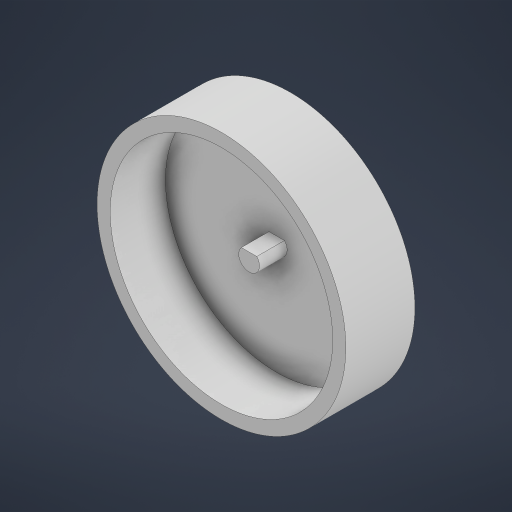
# Autodesk Inventor part: forma_do_kół
Saved by Autodesk Inventor 2023.4 (Build 274418000, 418)
## iProperties
Created: 2025-10-31
Part Number: forma_do_kół
Material: Ogólny
Document SubType Name: Modeling
Designer: Jakub Borsukiewicz
Density: 1 g/cm^3
Appearance: Domyślna
Author: Jakub Borsukiewicz
Autodesk Inventor part; units mm, degrees
ref_plane "YZ Plane" through (0, 0, 0) normal (1, 0, 0) x (0, 1, 0)
ref_plane "XZ Plane" through (0, 0, 0) normal (0, 1, 0) x (-1, 0, 0)
ref_plane "XY Plane" through (0, 0, 0) normal (0, 0, 1) x (1, 0, 0)
sketch "Szkic1" plane through (0, 0, 0) normal (0, 0, 1) x (1, 0, 0)
  circle A0 centre (0, 0) radius 18
  dimension "d0" = 36
  constraints: 1 centre point, 1 coincident
  measures "d0" diameter of A0
extrude "Wyciągnięcie proste1" add sketch "Szkic1" along normal blind 2
sketch "Szkic2" plane through (0, 0, 2) normal (0, 0, 1) x (1, 0, 0)
  circle A0 centre (0, 0) radius 1.5
  line L0 (0, 25.2) -> (0, -25.2) projected
  line L1 (-25.2, 0) -> (25.2, 0) projected
  line L2 (-1.118, 1) -> (1.118, 1)
  circle A1 centre (0, 0) radius 18 projected
  dimension "d3" = 3
  dimension "d4" = 1
  constraints: 2 end point, 2 point on circle, 1 centre point, 1 coincident, 1 horizontal
  measures "d3" diameter of A0
  measures "d4" distance between parallel lines of L1 L2
extrude "Wyciągnięcie proste2" add sketch "Szkic2" along normal blind 4 contours L1 L0 L2 A0 | A0 L0 L1 | A0 L1 L0 | L1 A0 L2 L0
sketch "Szkic3" plane through (0, 0, 2) normal (0, 0, 1) x (1, 0, 0)
  line L0 (-1.118, 1) -> (1.118, 1) projected
  arc A0 (-1.118, 1) -> (1.118, 1) centre (0, 0) ccw projected
  circle A1 centre (0, 0) radius 18 projected
  circle A2 centre (0, 0) radius 16.1
  dimension "d8" = 32.2
  constraints: 1 centre point, 1 coincident
  measures "d8" diameter of A2
extrude "Wyciągnięcie proste3" add sketch "Szkic3" along normal blind 8 contours A1
